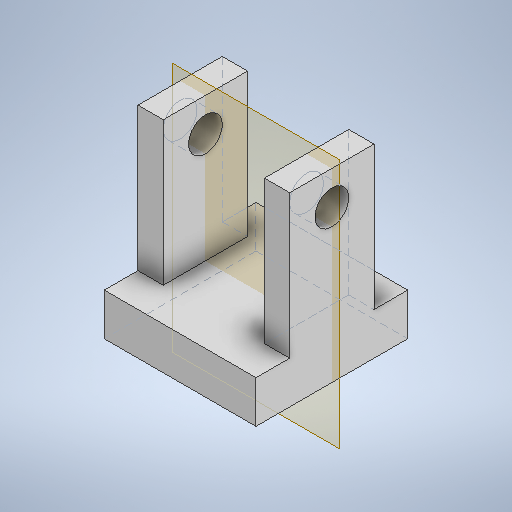
# Autodesk Inventor part: CT_01
Saved by Autodesk Inventor 2025.2 (Build 292293000, 293)
## iProperties
Created: 2024-12-05
Part Number: CT_01
Material: Generic
Document SubType Name: Modeling
Designer: hongquan
Density: 1 g/cm^3
Appearance: Default
Author: hongquan
Autodesk Inventor part; units mm, degrees
ref_plane "YZ Plane" through (0, 0, 0) normal (1, 0, 0) x (0, 1, 0)
ref_plane "XZ Plane" through (0, 0, 0) normal (0, 1, 0) x (-1, 0, 0)
sketch "Sketch1" plane through (0, 0, 0) normal (1, 0, 0) x (0, 1, 0)
  line L0 (0, 0) -> (90, 0)
  line L1 (90, 0) -> (90, -90)
  line L2 (90, -90) -> (0, -90)
  line L3 (0, -90) -> (0, 0)
  dimension "d0" = 90
  dimension "d1" = 90
  constraints: 8 end point, 2 parallel, 1 horizontal, 1 perpendicular
  measures "d0" distance of L2.end L0.start
  measures "d1" distance of L1.end L2.end
ref_plane "Work Plane1" through (0, 90, 0) normal (1, 0, 0) x (0, 1, 0)
sketch "Sketch2" plane through (0, 90, 0) normal (1, 0, 0) x (0, 1, 0)
  line L0 (20, -20) -> (-65, -20)
  line L1 (-65, -20) -> (-65, 0)
  line L2 (-65, 0) -> (-90, 0)
  line L3 (-90, 0) -> (-90, -90)
  line L4 (-90, -90) -> (-65, -90)
  line L5 (-65, -90) -> (-65, -70)
  line L6 (-65, -70) -> (20, -70)
  line L7 (20, -70) -> (20, -20)
  line L8 (0, -90) -> (0, 0) projected
  line L9 (0, 0) -> (0, -90)
  line L10 (-90, 0) -> (-90, -90) projected
  line L11 (0, -90) -> (-90, -90)
  line L12 (-90, -90) -> (-90, 0)
  line L13 (-90, 0) -> (0, 0)
  line L14 (0, -45) -> (-90, -45) construction
  circle A0 centre (0, -45) radius 10
  point P0 (20, -45)
  point P1 (-90, -45)
  point P2 (0, -70)
  point P3 (-65, 0)
  point P4 (0, -20)
  point P5 (0, -35)
  point P6 (0, -55)
  dimension "d4" = 90
  dimension "d7" = 50
  dimension "d10" = 20
  dimension "d11" = 90
  dimension "d13" = 25
  dimension "d14" = 25
  dimension "d27" = 110
  constraints: 26 end point, 7 perpendicular, 5 midpoint, 3 horizontal, 2 point on line, 2 vertical, 1 centre point, 1 coincident, 1 collinear
  measures "d4" distance of L2.end L3.end
  measures "d7" distance of L6.end L0.start
  measures "d10" diameter of A0
  measures "d11" distance from line of L3 A0.centre
  measures "d13" distance of L3.end L4.end
  measures "d14" distance of L2.end L1.end
  measures "d27" distance between parallel lines of L12 L7
ref_plane "Work Plane2" through (45, 110, -45) normal (0, 0, 1) x (1, 0, 0)
sketch "Sketch4" plane through (45, 110, -45) normal (0, 0, 1) x (1, 0, 0)
  line L0 (-90, 0) -> (0, 0) projected
  line L1 (-90, 0) -> (0, 0)
  line L2 (0, 0) -> (0, -110)
  line L3 (0, -110) -> (-90, -110)
  line L4 (-90, -110) -> (-90, 0)
  line L5 (-90, 0) -> (-75, 0)
  line L6 (-75, 0) -> (-15, 0)
  line L7 (-15, 0) -> (0, 0)
  line L8 (0, -110) -> (0, 0)
  line L9 (0, -110) -> (0, -85)
  line L10 (0, -85) -> (-90, -85)
  line L11 (-75, 0) -> (-75, -85)
  line L12 (-15, 0) -> (-15, -85)
  point P0 (-45, -110)
  dimension "d22" = 15
  dimension "d23" = 60
  dimension "d24" = 25
  dimension "d28" = 110
  constraints: 24 end point, 7 perpendicular, 6 point on line, 2 collinear
  measures "d22" distance of L0.start L5.end
  measures "d23" distance of L5.end L6.end
  measures "d24" distance of L2.end L9.end
  measures "d28" distance between parallel lines of L3 L0
extrude "Extrusion6" add sketch "Sketch2" along normal mid plane 90 contours L7 L6 L8 A0 L0 | L8 A0 L6 L5 L4 L3 L2 L1 L0
extrude "Extrusion7" cut sketch "Sketch4" along normal mid plane 90 contours L0 L12 L10 L11
body "Solid2"
